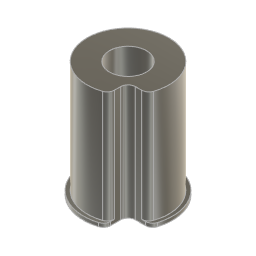
infinity_spool_core_parametric (Autodesk Fusion 360 design; units mm, degrees)
Autodesk Fusion 360 part; units mm, degrees
note: some values were not read from the file. Set by a fixed rule: which sketch regions a step uses.
sketch "Sketch1" plane through (0, 0, 0) normal (0, 0, 1) x (1, 0, 0) in component "Infinity Spool Core"
  circle A0 centre (0, 0) radius 5.1
  line L0 (4.975, 0) -> (2.4875, 4.3085)
  line L1 (2.4875, 4.3085) -> (-2.4875, 4.3085)
  line L2 (-2.4875, 4.3085) -> (-4.975, 0)
  line L3 (-4.975, 0) -> (-2.4875, -4.3085)
  line L4 (-2.4875, -4.3085) -> (2.4875, -4.3085)
  line L5 (2.4875, -4.3085) -> (4.975, 0)
  circle A1 centre (0, 0) radius 11.25
  circle A2 centre (0, 0) radius 12.25
  line L6 (5, -5) -> (5, -11.1831)
  line L7 (5, -5) -> (11.1831, -5)
  dimension "d66_1" = 10.2
  dimension "d68_1" = 4.975
  dimension "d69_1" = 22.5
  dimension "d70_1" = 1
  constraint coincident A0.centre A1.centre
  constraint coincident A2 L6.end
  constraint vertical L6
  constraint coincident A2 L7.end
  constraint perpendicular L6 L7
  measures "d66_1" diameter of A0
  measures "d68_1" distance of L0.start A0.centre
  measures "d69_1" diameter of A1
extrude "Extrude1" add sketch "Sketch1" along normal blind 31.75 contours A1 L6 L7 picked at (3.9544, -6.6084) in component "Infinity Spool Core"
extrude "Extrude2" add sketch "Sketch1" along normal blind 1 contours A1 A2 L6 L7 picked at (4.4871, -10.6551) in component "Infinity Spool Core"
fillet "Fillet1" radius 2 5 edges at (5, -10.0778, 16.375) (5, -5, 15.875) (10.0778, -5, 16.375) (5, -11.1831, 0.5) (11.1831, -5, 0.5) in component "Infinity Spool Core"
component "Infinity Spool Core" placed x (1, 0, 0) y (0, 1, 0) z (0, 0, 1) at (0, 0, 0)
equation "d69_1 = core_diameter - 0.5 mm"
equation "d71_1 = core_length - 0.25 mm"
equation "core_diameter = 23 mm"
equation "core_length = 32 mm"
named bodies: "infinity_spool_core"
